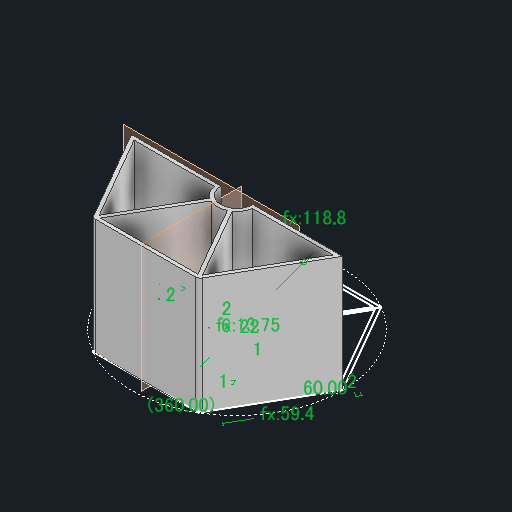
# Autodesk Inventor part: baicPart
Saved by Autodesk Inventor 2025.2 (Build 292293000, 293)
## iProperties
Company: FC-TORQUE
Created: 2025-03-14
Part Number: baicPart
Material: 一般
Document SubType Name: Modeling
Designer: Keito Tamura
Density: 1 g/cm^3
Appearance: 既定
Author: Keito Tamura
Autodesk Inventor part; units mm, degrees
ref_plane "XZ Plane" through (0, 0, 0) normal (0, 1, 0) x (-1, 0, 0)
ref_plane "XY Plane" through (0, 0, 0) normal (0, 0, 1) x (1, 0, 0)
sketch "スケッチ1" plane through (0, 0, 0) normal (0, 1, 0) x (-1, 0, 0)
  circle A0 centre (0, 0) radius 11
  circle A1 centre (0, 0) radius 59.4 construction
  line L0 (59.4, 0) -> (-59.4, 0)
  line L1 (-59.4, 0) -> (-29.7, 51.4419)
  line L2 (-59.4, 0) -> (0, 0) construction
  line L3 (-29.7, 51.4419) -> (0, 0)
  line L4 (-29.1226, 48.4419) -> (-1.7321, 1)
  line L5 (-56.5132, 1) -> (-1.7321, 1)
  line L6 (-29.1226, 48.4419) -> (-56.5132, 1)
  line L7 (-56.5132, -1) -> (-1.7321, -1)
  line L8 (-56.5132, -1) -> (-29.1226, -48.4419)
  line L9 (-29.1226, -48.4419) -> (-1.7321, -1)
  circle A2 centre (0, 0) radius 11
  line L10 (-59.4, 0) -> (0, 0)
  line L11 (-29.7, -51.4419) -> (-59.4, 0)
  line L12 (29.7, 51.4419) -> (-29.7, -51.4419)
  line L13 (-27.3906, -49.4419) -> (0, -2)
  line L14 (-27.3906, -49.4419) -> (27.3906, -49.4419)
  line L15 (27.3906, -49.4419) -> (0, -2)
  circle A3 centre (0, 0) radius 11
  line L16 (-29.7, -51.4419) -> (0, 0)
  line L17 (29.7, -51.4419) -> (-29.7, -51.4419)
  line L18 (-29.7, 51.4419) -> (29.7, -51.4419)
  line L19 (29.1226, -48.4419) -> (1.7321, -1)
  line L20 (29.1226, -48.4419) -> (56.5132, -1)
  line L21 (56.5132, -1) -> (1.7321, -1)
  circle A4 centre (0, 0) radius 11
  line L22 (29.7, -51.4419) -> (0, 0)
  line L23 (59.4, 0) -> (29.7, -51.4419)
  line L24 (-59.4, 0) -> (59.4, 0)
  line L25 (56.5132, 1) -> (1.7321, 1)
  line L26 (56.5132, 1) -> (29.1226, 48.4419)
  line L27 (29.1226, 48.4419) -> (1.7321, 1)
  circle A5 centre (0, 0) radius 11
  line L28 (59.4, 0) -> (0, 0)
  line L29 (29.7, 51.4419) -> (59.4, 0)
  line L30 (-29.7, -51.4419) -> (29.7, 51.4419)
  line L31 (27.3906, 49.4419) -> (0, 2)
  line L32 (27.3906, 49.4419) -> (-27.3906, 49.4419)
  line L33 (-27.3906, 49.4419) -> (0, 2)
  circle A6 centre (0, 0) radius 11
  line L34 (29.7, 51.4419) -> (0, 0)
  line L35 (-29.7, 51.4419) -> (29.7, 51.4419)
  line L36 (29.7, -51.4419) -> (-29.7, 51.4419)
  circle A7 centre (0, 0) radius 9
  circle A8 centre (5.9815, 3.3893) radius 3
  circle A9 centre (0, 0) radius 6.875 construction
  line L37 (55.9359, 2) -> (-55.9359, 2)
  point P0 (-6.3433, 8.9868)
  point P1 (-10.9545, 1)
  point P2 (10.9545, 1)
  point P3 (6.3433, 8.9868)
  point P4 (-6.3433, -8.9868)
  point P5 (-10.9545, -1)
  point P6 (4.6112, -9.9868)
  point P7 (-4.6112, -9.9868)
  point P8 (10.9545, -1)
  point P9 (6.3433, -8.9868)
  point P10 (4.6112, 9.9868)
  point P11 (-4.6112, 9.9868)
  point P12 (-29.7, 51.4419)
  point P13 (-59.4, 0)
  point P14 (-29.7, -51.4419)
  point P15 (29.7, -51.4419)
  point P16 (59.4, 0)
  point P17 (29.7, 51.4419)
  point P18 (-9, 0)
  point P19 (9, 0)
  point P20 (-8.9443, 1)
  point P21 (-8.775, 2)
  point P22 (8.775, 2)
  point P23 (8.9443, 1)
  dimension "d17" = 13.75
  dimension "d0" = 22
  dimension "d1" = 118.8
  dimension "d2" = 60
  dimension "d3" = 59.4
  dimension "d4" = 1
  dimension "d5" = 1
  dimension "d6" = 2
  dimension "d9" = 360
  dimension "d11" = 2
  dimension "d16" = 6
  dimension "d23" = 2
  constraints: 76 end point, 9 centre point, 5 coincident, 3 horizontal, 2 point on circle, 2 point on line, 1 equal length, 1 midpoint, 1 parallel, 100 other
  measures "d0" diameter of A0
  measures "d1" diameter of A1
  measures "d2" angle of L2 L1
  measures "d3" distance of L0.end L1.end
  measures "d4" distance between parallel lines of L3 L4
  measures "d5" distance between parallel lines of L0 L5
  measures "d6" distance between parallel lines of L6 L1
  measures "d11" radial gap between concentric circles of A0 A7
  measures "d16" diameter of A8
  measures "d23" distance between parallel lines of L37 L0
extrude "押し出し1" add sketch "スケッチ1" along normal blind 65.34 contours L0 A7 L25 A0 | L0 L23 L18 A0 L19 L20 L21 | A0 L25 L26 L27 L12 L29 L0 | A0 L21 A7 L0 | L25 A7 L37 A0 | A0 L19 A7 L21 | L37 A7 A8 L27 A0 | A0 L18 A7 L19 | L17 L12 A0 L13 L14 L15 L18 | L12 A0 L31 L32 L33 L3 L35 | L27 A7 L12 A0 | A0 L15 A7 L18 | L11 L0 A0 L7 L8 L9 L12 | L12 A7 L31 A0 | L3 A0 L4 L6 L5 L0 L1 | A7 L7 A0 L0 | L0 A0 L5 A7 | A7 L13 A0 L12 | L12 A0 L9 A7 | A7 A8 | A0 L13 A7 L15 | L31 A7 L33 A0 | L3 A7 L4 A0 | A0 L33 A7 L3 | L5 A0 L37 A7 | A7 L9 A0 L7 | L4 A7 L37 A0
extrude "押し出し2" add sketch "スケッチ1" along normal blind 2 contours A0 L37 L26 L25 | L0 L12 L37 L27 L25 A8 A7 | A0 L27 L26 L37 | L25 A8 L37 A7 | L0 A7 L5 L4 L37 L3 | L3 L37 L12 | L37 A8 A7 | A8 L25 | L25 A8 L37 | L37 L4 A7 L3 | L3 A7 L33 L37 | L37 L31 A7 L12 | L12 A7 L27 A8 L37 | A7 A8 L27 | A8 L37 L27 A7 | L25 L27 L37 A8 | A0 L33 L32 L31 | A7 L37 L4 L5 | L33 A7 L31 | L37 A7 L4 | L27 A8 L37 | L27 A8 | A0 L37 L6 L4 | L5 L6 L37 A0
ref_plane "作業平面1" through (-56.5132, 65.34, 0) normal (0, 0, 1) x (1, 0, 0)
split "分割1" plane through (-56.5132, 65.34, 0) removes the side toward (0, 0, -1)
extrude "押し出し4" add sketch "スケッチ1" along normal blind 65.34 contours L25 A7 L37 A0 | A0 L37 L26 L25 | L5 A0 L37 A7 | L5 L6 L37 A0
sketch "スケッチ2" plane through (0, 2, 0) normal (0, 1, 0) x (1, 0, 0)
  circle A0 centre (0, -42.9469) radius 2
  circle A1 centre (0, -19.1869) radius 2
  line L0 (-2, -42.9469) -> (2, -42.9469) construction
  line L1 (2, -42.9469) -> (2, -19.1869)
  line L2 (2, -19.1869) -> (-2, -19.1869) construction
  line L3 (-2, -19.1869) -> (-2, -42.9469)
  point P0 (0, 0)
  point P1 (2, -42.9469)
  point P2 (-2, -19.1869)
  point P3 (0, -19.1869)
  point P4 (0, -42.9469)
  dimension "d26" = 4
  dimension "d27" = 4
  dimension "d50" = 23.76
  constraints: 8 end point, 2 midpoint, 2 parallel, 1 horizontal, 1 perpendicular, 6 other
  measures "d50" distance of point (0, -19.187) point (0, -42.947)
extrude "押し出し5" cut sketch "スケッチ2" against normal blind 1
pattern_circular "円形状パターン2" count 3 over 120 about axis through (0, 0, 0) along (0, 1, 0) of "押し出し5" both ways yes
sketch "スケッチ3" plane through (0, 2, 0) normal (0, 1, 0) x (1, 0, 0)
  circle A0 centre (-17.5202, -37.3458) radius 1
  line L0 (-17.5202, -37.3458) -> (-8.8206, -22.2777)
  line L1 (-27.3906, -49.4419) -> (-4.6112, -9.9868) projected
  circle A1 centre (-8.8206, -22.2777) radius 1
  line L2 (-18.3862, -36.8458) -> (-9.6866, -21.7777)
  line L3 (-16.9447, -38.1637) -> (-7.9545, -22.7777)
  point P0 (0, 0)
  dimension "d33" = 2
  dimension "d34" = 2
  dimension "d35" = 2.5
  dimension "d51" = 17.82
  constraints: 6 end point, 4 point on circle, 2 centre point, 1 coincident, 1 parallel, 1 tangent
  measures "d33" diameter of A0
  measures "d34" diameter of A1
  measures "d35" distance between parallel lines of L1 L0
  measures "d51" distance of L3.start L3.end
extrude "押し出し6" cut sketch "スケッチ3" against normal through all contours A0 L3 | L2 A1 L0 A0 | L0 A1 L3 A0 | A1 picked at (-17.2385, -37.0808)
pattern_circular "円形状パターン3" count 2 over 60 about axis through (0, 0, 0) along (0, 1, 0) of "押し出し6"
mirror "ミラー1" about plane through (0, 0, 0) normal (1, 0, 0) of "押し出し6", "円形状パターン3"
fillet "フィレット1" radius 3 2 edges at (29.7, 32.67, 51.4419) (-29.7, 32.67, 51.4419)
fillet "フィレット3" radius 2 12 edges at (42.5293, 2, 25.221) (17.733, 2, 28.7144) (33.3763, 2, 2) (16.0009, 2, 29.7144) (0, 2, 11) (-16.0009, 2, 29.7144) (0, 2, 49.4419) (9.2639, 2, 5.9313) (-17.733, 2, 28.7144) (-42.5293, 2, 25.221) (-33.3763, 2, 2) (-9.2639, 2, 5.9313)
sketch "スケッチ6" plane through (0, 2, 0) normal (0, 1, 0) x (1, 0, 0)
  point P0 (0, 0)
sketch "スケッチ7" plane through (0, 2, 0) normal (0, 1, 0) x (1, 0, 0)
  line L0 (18.3862, -37.8458) -> (23.9265, -47.4419) projected
  arc A0 (16.9447, -38.1637) -> (18.3862, -37.8458) centre (17.5202, -37.3458) ccw projected
  line L1 (16.9447, -38.1637) -> (7.9545, -22.7777) projected
  arc A1 (8.8206, -21.2777) -> (7.9545, -22.7777) centre (8.8206, -22.2777) ccw projected
  line L2 (3.7265, -12.4545) -> (8.8206, -21.2777) projected
  arc A2 (-3.7265, -12.4545) -> (3.7265, -12.4545) centre (0, 0) ccw projected
  line L3 (-8.8206, -21.2777) -> (-3.7265, -12.4545) projected
  arc A3 (-7.9545, -22.7777) -> (-8.8206, -21.2777) centre (-8.8206, -22.2777) ccw projected
  line L4 (-7.9545, -22.7777) -> (-16.9447, -38.1637) projected
  arc A4 (-18.3862, -37.8458) -> (-16.9447, -38.1637) centre (-17.5202, -37.3458) ccw projected
  line L5 (-23.9265, -47.4419) -> (-18.3862, -37.8458) projected
  line L6 (23.9265, -47.4419) -> (-23.9265, -47.4419) projected
  arc A5 (2, -19.1869) -> (-2, -19.1869) centre (0, -19.1869) ccw projected
  line L7 (2, -19.1869) -> (2, -42.9469) projected
  arc A6 (-2, -42.9469) -> (2, -42.9469) centre (0, -42.9469) ccw projected
  line L8 (-2, -42.9469) -> (-2, -19.1869) projected
  arc A7 (-4.6112, -9.9868) -> (4.6112, -9.9868) centre (0, 0) ccw projected
  circle A8 centre (0, 0) radius 39.204
  circle A9 centre (-9.4843, -38.0395) radius 3
  line L9 (-9.4843, -38.0395) -> (0, 0)
  line L10 (83.16, 0) -> (-83.16, 0) projected
  dimension "d53" = 78.408
  dimension "d54" = 6
  dimension "d55" = 76
  constraints: 2 end point, 1 centre point, 1 coincident, 3 other
  measures "d54" diameter of A9
  measures "d55" angle of L10 L9
extrude "押し出し9" cut sketch "スケッチ7" against normal through all contours A9 A8 | A8 L9 A9 | A9 L9 A8
pattern_circular "円形状パターン4" count 3 over 120 about axis through (0, 0, 0) along (0, 1, 0) of "押し出し9" both ways yes
mirror "ミラー2" about plane through (0, 0, 0) normal (1, 0, 0) of "押し出し9", "円形状パターン4"
sketch "スケッチ8" plane through (0, 2, 0) normal (0, 1, 0) x (1, 0, 0)
  line L0 (55.9359, -2) -> (10.8167, -2) projected
  line L1 (30.9758, -2) -> (28.9758, -2)
  line L2 (28.9758, -2) -> (28.9758, -11.4062)
  line L3 (28.9758, -11.4062) -> (30.9758, -11.4062)
  line L4 (30.9758, -11.4062) -> (30.9758, -2)
  point P0 (0, 0)
  dimension "d61" = 2
  constraints: 8 end point, 2 parallel, 1 horizontal, 1 perpendicular, 1 point on line
  measures "d61" distance of L3.end L2.end
extrude "押し出し10" add sketch "スケッチ8" along normal blind 30
mirror "ミラー3" about plane through (0, 0, 0) normal (1, 0, 0) of "押し出し10"
equation "\"d17\" = 0.625 * d0"
equation "\"d1\" = 5.4 * d0"
equation "\"d3\" = 0.5 * d1"
equation "\"d12\" = 1.1 * d3"
equation "\"d24\" = 1.1 * d3"
equation "\"d50\" = 0.4 * d3"
equation "\"d33\" = d34"
equation "\"d51\" = 0.3 * d3"
equation "\"d53\" = 0.66 * d1"
